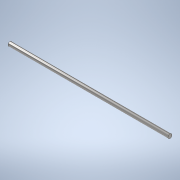
# Autodesk Inventor part: Part9
Saved by Autodesk Inventor 2022 (Build 260153070, 153G)
## iProperties
Created: 2021-07-07
Part Number: Part9
Material: Steel, Alloy
Document SubType Name: Modeling
Designer: sachin
Density: 7.73 g/cm^3
Appearance: Semi-Polished
Author: sachin
Autodesk Inventor part; units mm, degrees
ref_plane "YZ Plane" through (0, 0, 0) normal (1, 0, 0) x (0, 1, 0)
ref_plane "XZ Plane" through (0, 0, 0) normal (0, 1, 0) x (-1, 0, 0)
ref_plane "XY Plane" through (0, 0, 0) normal (0, 0, 1) x (1, 0, 0)
sketch "Sketch1" plane through (0, 0, 0) normal (1, 0, 0) x (0, 1, 0)
  circle A0 centre (15.789, 26.9983) radius 5.08
  point P0 (0, 0)
  dimension "d0" = 10.16
  dimension "d0" = 10.16
  constraints: 1 centre point
  measures "d0" diameter of A0
extrude "Extrusion1" add sketch "Sketch1" along normal blind 400
body "Solid1"
